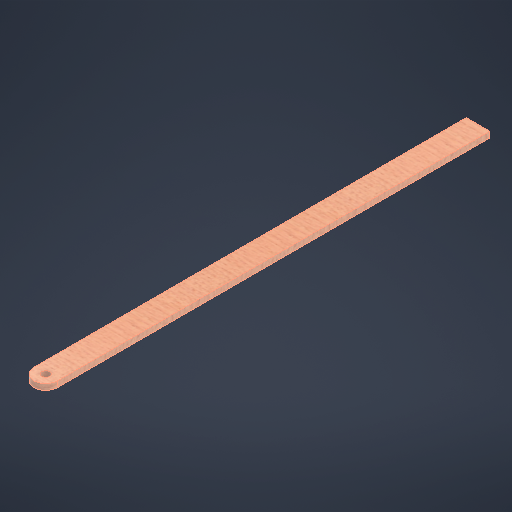
# Autodesk Inventor part: COUNTERWEIGHT_OUTSIDE_ARM,TREBUCHET
Saved by Autodesk Inventor 2026.2 (Build 302298010, 298A)
## iProperties
Created: 2026-02-12
Part Number: COUNTERWEIGHT_OUTSIDE_ARM,TREBUCHET
Material: Wood (Oak)
Document SubType Name: Modeling
Designer: 4aida
Density: 0.76 g/cm^3
Appearance: White Oak - Natural Medium Gloss
Author: 4aida
Autodesk Inventor part; units mm, degrees
ref_plane "YZ Plane" through (0, 0, 0) normal (1, 0, 0) x (0, 1, 0)
ref_plane "XZ Plane" through (0, 0, 0) normal (0, 1, 0) x (-1, 0, 0)
ref_plane "XY Plane" through (0, 0, 0) normal (0, 0, 1) x (1, 0, 0)
sketch "Sketch1" plane through (0, 0, 0) normal (0, 1, 0) x (-1, 0, 0)
  line L0 (-19.05, -914.4) -> (19.05, -914.4)
  line L1 (19.05, -914.4) -> (19.05, 914.4)
  line L2 (19.05, 914.4) -> (-19.05, 914.4)
  line L3 (-19.05, 914.4) -> (-19.05, -914.4)
  line L4 (-19.05, -914.4) -> (19.05, 914.4) construction
  line L5 (19.05, -914.4) -> (-19.05, 914.4) construction
  point P0 (0, 0)
  dimension "d0" = 38.1
  dimension "d1" = 1828.8
  constraints: 12 end point, 2 midpoint, 2 parallel, 1 horizontal, 1 perpendicular
  measures "d0" distance of L2.end L1.end
  measures "d1" distance of L1.end L0.end
extrude "Extrusion1" add sketch "Sketch1" along normal mid plane 9.525
sketch "Sketch2" plane through (0, 4.7625, 0) normal (0, 1, 0) x (1, 0, 0)
  circle A0 centre (0, -895.35) radius 6.35
  line L0 (-19.05, 914.4) -> (-19.05, -914.4) projected
  line L1 (19.05, -914.4) -> (19.05, 914.4) projected
  arc A1 (-19.05, -895.35) -> (19.05, -895.35) centre (0, -895.35) ccw
  line L2 (-19.05, -914.4) -> (19.05, -914.4) projected
  line L3 (-19.05, -195.35) -> (19.05, -195.35)
  point P0 (0, 0)
  point P1 (0, -914.4)
  dimension "d4" = 12.7
  dimension "d5" = 700
  constraints: 4 point on line, 3 point on circle, 2 centre point, 2 end point, 1 coincident, 1 midpoint, 1 perpendicular, 1 tangent
  measures "d4" diameter of A0
  measures "d5" distance from line of L3 A0.centre
extrude "Extrusion2" cut sketch "Sketch2" against normal through all contours L3 L1 A1 L0 keep common part
body "Solid1"
